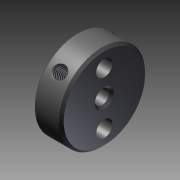
# Autodesk Inventor part: SSCTN3b
Saved by Autodesk Inventor 2015 (Build 190159000, 159)
## iProperties
Category: PARTsolutions
Company: MISUMI
Created: 2015-06-23
Part Number: SSCTN3b
Catalog Web Link: www.cadenas.de
Description: SCTN, PSCTN, SSCTN, SCTW, PSCTW, SSCTW-b-Shaft Collars - With Holes/Threaded - 2 Hole
Vendor: MISUMI
Document SubType Name: Modeling
Designer: PARTuser1
Manufacturer: MISUMI
Mass: 1.28428 g
Surface Area: 10.4132 cm^2
Volume: 1.28428 cm^3
Density: 1 g/cm^3
Material: 一般
Appearance: PSOLRGB-192-192-192
PSOL_IDENT_0: {$CADENAS_DATA\23d-libs\misumi\metric\03_set_collars\sctn_b.prj},199 {VTYP=3D},{NB=SSCTN3b},{LINA=SS
PSOL_IDENT_1: CTN3b},{NN=SCTN, PSCTN, SSCTN, SCTW, PSCTW, SSCTW-b},{DATE=22.04.2015 10:30:22},{GEOMDATE=21.01.2010
PSOL_IDENT_2: 10:30:00},{VERSION=},{LINEID=10},{LINESUBID=-1},{WBVAR=TS,MAT,ST}  {NB=SSCTN3b},{LINA=SSCTN3b},{KT=
PSOL_IDENT_3: DUMMY},{PN=SSCTN3},{TS=N},{TSA= 'N' , 'Hole' , 'W' , 'Threaded Hole' },{TYPE=SSCTN},{MAT=304},{ST=-}
PSOL_IDENT_4: ,{AC=Set Screws 2 Pcs. (304 Stainless Steel) },{D=3},{B=6},{D1=18},{S=3.4},{P=11},{M=M3x3},{THMD=3},
PSOL_IDENT_5: {THDMIN=2.459},{M1=M3},{M1NDM=3},{C=0.5},{ST0='-','-'},{L=3}
SUPPLIER: MISUMI
ARTICLENO: SSCTN3b
BOMINFO: SSCTN3b
CREATOR: CADENAS GmbH
Title: SSCTN3b
Author: Cadenas PARTsolutions
Comments: Shaft Collars - With Holes/Threaded - 2 Hole
Autodesk Inventor part; units mm, degrees
sketch "Sketch_1" plane through (0, 0, 0) normal (0, 0, 1) x (1, 0, 0)
  line L0 (0, 0) -> (-3, 0)
  line L1 (-3, 8.5) -> (-3, 2)
  line L2 (-3, 2) -> (-2.5, 1.5)
  line L3 (-2.5, 1.5) -> (2.5, 1.5)
  line L4 (2.5, 1.5) -> (3, 2)
  line L5 (3, 2) -> (3, 8.5)
  line L6 (3, 8.5) -> (2.5, 9)
  line L7 (2.5, 9) -> (-2.5, 9)
  line L8 (-2.5, 9) -> (-3, 8.5)
  constraints: 18 end point
revolve "Revolution1" add sketch "Sketch_1" angle 360 about axis through (0, 0, 0) along (1, 0, 0)
sketch "Sketch_2" plane through (0, 0, 0) normal (1, 0, 0) x (0, 1, 0)
  line L0 (7.0004, 7.0004) -> (0.4243, 0.4243)
  line L1 (0.4243, 0.4243) -> (-0.6364, 1.4849)
  line L2 (-0.6364, 1.4849) -> (0, 2.1213)
  line L3 (0, 2.1213) -> (0.3825, 2.1213)
  line L4 (0.3825, 2.1213) -> (5.3033, 7.0421)
  line L5 (5.3033, 7.0421) -> (5.3033, 7.4246)
  line L6 (5.3033, 7.4246) -> (5.9397, 8.061)
  line L7 (5.9397, 8.061) -> (7.0004, 7.0004)
  line L8 (7.0004, 7.0004) -> (0.4243, 0.4243)
  constraints: 18 end point
revolve "Revolution2" cut sketch "Sketch_2" angle 360 about axis through (0, 7.0004, 7.0004) along (0, 0.7071068, 0.7071068)
thread "Thread1" size "M3x0.5" class "6H" standard "ISO Metric profile" full length
sketch "Sketch_3" plane through (0, 0, 0) normal (1, 0, 0) x (0, 1, 0)
  line L0 (-7.0004, 7.0004) -> (-0.4243, 0.4243)
  line L1 (-0.4243, 0.4243) -> (-1.4849, -0.6364)
  line L2 (-1.4849, -0.6364) -> (-2.1213, 0)
  line L3 (-2.1213, 0) -> (-2.1213, 0.3825)
  line L4 (-2.1213, 0.3825) -> (-7.0421, 5.3033)
  line L5 (-7.0421, 5.3033) -> (-7.4246, 5.3033)
  line L6 (-7.4246, 5.3033) -> (-8.061, 5.9397)
  line L7 (-8.061, 5.9397) -> (-7.0004, 7.0004)
  line L8 (-7.0004, 7.0004) -> (-0.4243, 0.4243)
  constraints: 18 end point
revolve "Revolution3" cut sketch "Sketch_3" angle 360 about axis through (0, -7.0004, 7.0004) along (0, -0.7071068, 0.7071068)
thread "Thread2" size "M3x0.5" class "6H" standard "ISO Metric profile" full length
sketch "Sketch_6" plane through (0, 0, 0) normal (1, 0, 0) x (0, 1, 0)
  circle A0 centre (0, -5.5) radius 1.7
  constraints: 1 centre point
extrude "Extrusion1" cut sketch "Sketch_6" along normal mid plane 12
sketch "Sketch_7" plane through (0, 0, 0) normal (1, 0, 0) x (0, 1, 0)
  circle A0 centre (0, 5.5) radius 1.7
  constraints: 1 centre point
extrude "Extrusion2" cut sketch "Sketch_7" along normal mid plane 12
ref_plane "body_set_h_XY" through (0, -6.364, 6.364) normal (0, 0.7071068, -0.7071068) x (1, 0, 0)
ref_plane "body_set_h_YZ" through (0, -6.364, 6.364) normal (1, 0, 0) x (0, -0.7071068, -0.7071068)
ref_plane "body_set_h_ZX" through (0, -6.364, 6.364) normal (0, -0.7071068, -0.7071068) x (0, 0.7071068, -0.7071068)
ref_plane "body_set_v_XY" through (0, 6.364, 6.364) normal (0, 0.7071068, 0.7071068) x (1, 0, 0)
ref_plane "body_set_v_YZ" through (0, 6.364, 6.364) normal (1, 0, 0) x (0, 0.7071068, -0.7071068)
ref_plane "body_set_v_ZX" through (0, 6.364, 6.364) normal (0, 0.7071068, -0.7071068) x (0, 0.7071068, 0.7071068)
body "Solid1"
